Autodesk Inventor part; units mm, degrees
(part 5 of 5)
  arc A349 (-28.421, 226.0743) -> (-28.921, 225.5743) centre (-28.421, 225.5743) ccw
  arc A350 (-15.421, 212.0743) -> (-14.921, 212.5743) centre (-15.421, 212.5743) ccw
  arc A351 (-14.921, 225.5743) -> (-15.421, 226.0742) centre (-15.421, 225.5743) ccw
  line L356 (-28.921, 236.3868) -> (-28.921, 249.3868)
  line L357 (-14.921, 236.3868) -> (-14.921, 249.3868)
  line L358 (-28.421, 235.8868) -> (-15.421, 235.8868)
  line L359 (-28.421, 249.8868) -> (-15.421, 249.8867)
  arc A352 (-28.921, 236.3868) -> (-28.421, 235.8868) centre (-28.421, 236.3868) ccw
  arc A353 (-28.421, 249.8868) -> (-28.921, 249.3868) centre (-28.421, 249.3868) ccw
  arc A354 (-15.421, 235.8868) -> (-14.921, 236.3868) centre (-15.421, 236.3867) ccw
  arc A355 (-14.921, 249.3868) -> (-15.421, 249.8867) centre (-15.421, 249.3867) ccw
  line L360 (-28.921, 260.1993) -> (-28.921, 273.1993)
  line L361 (-14.921, 260.1992) -> (-14.921, 273.1993)
  line L362 (-28.421, 259.6993) -> (-15.421, 259.6993)
  line L363 (-28.421, 273.6992) -> (-15.421, 273.6992)
  arc A356 (-28.921, 260.1993) -> (-28.421, 259.6993) centre (-28.421, 260.1993) ccw
  arc A357 (-28.421, 273.6992) -> (-28.921, 273.1993) centre (-28.421, 273.1993) ccw
  arc A358 (-15.421, 259.6993) -> (-14.921, 260.1992) centre (-15.421, 260.1993) ccw
  arc A359 (-14.921, 273.1993) -> (-15.421, 273.6992) centre (-15.421, 273.1993) ccw
  line L364 (-28.921, 284.0118) -> (-28.921, 297.0118)
  line L365 (-14.921, 284.0118) -> (-14.921, 297.0118)
  line L366 (-28.421, 283.5118) -> (-15.421, 283.5118)
  line L367 (-28.421, 297.5118) -> (-15.421, 297.5118)
  arc A360 (-28.921, 284.0118) -> (-28.421, 283.5117) centre (-28.421, 284.0118) ccw
  arc A361 (-28.421, 297.5118) -> (-28.921, 297.0118) centre (-28.421, 297.0117) ccw
  arc A362 (-15.421, 283.5118) -> (-14.921, 284.0117) centre (-15.421, 284.0118) ccw
  arc A363 (-14.921, 297.0118) -> (-15.421, 297.5118) centre (-15.421, 297.0118) ccw
  line L368 (-28.921, 310.2055) -> (-28.921, 323.2055)
  line L369 (-14.921, 310.2055) -> (-14.921, 323.2055)
  line L370 (-28.421, 309.7055) -> (-15.421, 309.7055)
  line L371 (-28.421, 323.7055) -> (-15.421, 323.7055)
  arc A364 (-28.921, 310.2055) -> (-28.421, 309.7055) centre (-28.421, 310.2055) ccw
  arc A365 (-28.421, 323.7055) -> (-28.921, 323.2055) centre (-28.421, 323.2055) ccw
  arc A366 (-15.421, 309.7055) -> (-14.921, 310.2055) centre (-15.421, 310.2055) ccw
  arc A367 (-14.921, 323.2055) -> (-15.421, 323.7055) centre (-15.421, 323.2055) ccw
  line L372 (-28.921, 329.2555) -> (-28.921, 342.2555)
  line L373 (-14.921, 329.2555) -> (-14.921, 342.2555)
  line L374 (-28.421, 328.7555) -> (-15.421, 328.7555)
  line L375 (-28.421, 342.7555) -> (-15.421, 342.7555)
  arc A368 (-28.921, 329.2555) -> (-28.421, 328.7555) centre (-28.421, 329.2555) ccw
  arc A369 (-28.421, 342.7555) -> (-28.921, 342.2555) centre (-28.421, 342.2555) ccw
  arc A370 (-15.421, 328.7555) -> (-14.921, 329.2555) centre (-15.421, 329.2555) ccw
  arc A371 (-14.921, 342.2555) -> (-15.421, 342.7555) centre (-15.421, 342.2555) ccw
  line L376 (-28.921, 348.3055) -> (-28.921, 361.3055)
  line L377 (-14.921, 348.3055) -> (-14.921, 361.3055)
  line L378 (-28.421, 347.8055) -> (-15.421, 347.8055)
  line L379 (-28.421, 361.8055) -> (-15.421, 361.8055)
  arc A372 (-28.921, 348.3055) -> (-28.421, 347.8055) centre (-28.421, 348.3055) ccw
  arc A373 (-28.421, 361.8055) -> (-28.921, 361.3055) centre (-28.421, 361.3055) ccw
  arc A374 (-15.421, 347.8055) -> (-14.921, 348.3055) centre (-15.421, 348.3055) ccw
  arc A375 (-14.921, 361.3055) -> (-15.421, 361.8055) centre (-15.421, 361.3055) ccw
  line L380 (-12.396, 16.668) -> (-12.396, 364.3305)
  line L381 (-131.4585, 16.668) -> (-131.4585, 364.3305)
  line L382 (-12.396, 16.668) -> (-131.4585, 16.668)
  line L383 (-12.396, 364.3305) -> (-131.4585, 364.3305)
  point P0 (-71.9272, 364.3305)
  point P1 (-14.921, 28.5742)
  point P2 (-47.471, 269.2243)
  point P3 (-34.471, 269.2242)
  point P4 (-33.971, 269.7243)
  point P5 (-33.971, 282.7243)
  point P6 (-34.471, 283.2243)
  point P7 (-47.471, 283.2243)
  point P8 (-47.971, 282.7243)
  point P9 (-47.971, 269.7243)
  point P10 (-46.471, 260.7863)
  point P11 (-31.971, 261.2863)
  point P12 (-31.971, 267.2863)
  point P13 (-32.471, 267.7862)
  point P14 (-46.471, 267.7863)
  point P15 (-46.971, 267.2863)
  point P16 (-46.971, 261.2863)
  point P17 (-31.971, 285.1623)
  point P18 (-31.971, 291.1622)
  point P19 (-32.471, 291.6623)
  point P20 (-46.971, 285.1623)
  point P21 (-47.471, 328.7555)
  point P22 (-33.971, 329.2555)
  point P23 (-33.971, 342.2555)
  point P24 (-34.471, 342.7555)
  point P25 (-47.471, 342.7555)
  point P26 (-47.971, 342.2555)
  point P27 (-47.971, 329.2555)
  point P28 (-66.521, 273.9868)
  point P29 (-53.021, 274.4868)
  point P30 (-53.521, 287.9868)
  point P31 (-51.521, 265.5487)
  point P32 (-66.021, 266.0488)
  point P33 (-65.521, 289.4248)
  point P34 (-51.521, 289.4248)
  point P35 (-51.021, 295.9248)
  point P36 (-65.521, 296.4248)
  point P37 (-28.421, 259.6993)
  point P38 (-15.421, 259.6993)
  point P39 (-14.921, 273.1993)
  point P40 (-15.421, 273.6992)
  point P41 (-28.421, 273.6992)
  point P42 (-28.921, 273.1993)
  point P43 (-28.921, 260.1993)
  point P44 (-28.421, 283.5118)
  point P45 (-15.421, 283.5118)
  point P46 (-14.921, 297.0118)
  point P47 (-15.421, 297.5118)
  point P48 (-28.921, 297.0118)
  point P49 (-28.921, 284.0118)
  point P50 (-28.421, 309.7055)
  point P51 (-15.421, 309.7055)
  point P52 (-14.921, 310.2055)
  point P53 (-14.921, 323.2055)
  point P54 (-15.421, 323.7055)
  point P55 (-28.421, 323.7055)
  point P56 (-28.921, 323.2055)
  point P57 (-28.921, 310.2055)
  point P58 (-28.421, 328.7555)
  point P59 (-15.421, 328.7555)
  point P60 (-14.921, 329.2555)
  point P61 (-14.921, 342.2555)
  point P62 (-15.421, 342.7555)
  point P63 (-28.421, 342.7555)
  point P64 (-28.921, 342.2555)
  point P65 (-28.921, 329.2555)
  point P66 (-28.421, 347.8055)
  point P67 (-15.421, 347.8055)
  point P68 (-14.921, 348.3055)
  point P69 (-14.921, 361.3055)
  point P70 (-15.421, 361.8055)
  point P71 (-28.421, 361.8055)
  point P72 (-28.921, 361.3055)
  point P73 (-28.921, 348.3055)
  point P74 (-115.4335, 266.843)
  point P75 (-115.4335, 285.893)
  point P76 (-115.4335, 299.893)
  point P77 (-104.621, 276.368)
  point P78 (-91.621, 276.368)
  point P79 (-91.121, 289.868)
  point P80 (-104.621, 290.368)
  point P81 (-105.121, 289.868)
  point P82 (-105.121, 276.868)
  point P83 (-89.621, 267.93)
  point P84 (-89.121, 268.43)
  point P85 (-89.121, 274.43)
  point P86 (-104.121, 274.43)
  point P87 (-104.121, 268.43)
  point P88 (-89.621, 298.806)
  point P89 (-104.121, 298.306)
  point P90 (-104.621, 309.7055)
  point P91 (-91.621, 309.7055)
  point P92 (-91.121, 310.2055)
  point P93 (-91.121, 323.2055)
  point P94 (-91.621, 323.7055)
  point P95 (-91.121, 329.2555)
  point P96 (-91.121, 342.2555)
  point P97 (-91.621, 342.7555)
  point P98 (-104.621, 342.7555)
  point P99 (-105.121, 342.2555)
  point P100 (-105.121, 329.2555)
  point P101 (-104.621, 347.8055)
  point P102 (-91.621, 347.8055)
  point P103 (-91.121, 348.3055)
  point P104 (-91.121, 361.3055)
  point P105 (-91.621, 361.8055)
  point P106 (-104.621, 361.8055)
  point P107 (-105.121, 348.3055)
  point P108 (-85.571, 257.318)
  point P109 (-72.071, 257.818)
  point P110 (-72.071, 270.818)
  point P111 (-86.071, 270.818)
  point P112 (-86.071, 257.818)
  point P113 (-72.571, 281.1305)
  point P114 (-72.071, 281.6305)
  point P115 (-86.071, 281.6305)
  point P116 (-85.571, 309.7055)
  point P117 (-72.071, 310.2055)
  point P118 (-72.571, 323.7055)
  point P119 (-85.571, 323.7055)
  point P120 (-85.571, 328.7555)
  point P121 (-72.071, 329.2555)
  point P122 (-72.571, 342.7555)
  point P123 (-86.071, 342.2555)
  point P124 (-86.071, 329.2555)
  point P125 (-72.071, 348.3055)
  point P126 (-85.571, 361.8055)
  point P127 (-86.071, 361.3055)
  point P128 (-86.071, 348.3055)
  point P129 (-47.471, 195.4055)
  point P130 (-34.471, 195.4055)
  point P131 (-33.971, 195.9055)
  point P132 (-33.971, 208.9055)
  point P133 (-34.471, 209.4055)
  point P134 (-47.471, 209.4055)
  point P135 (-47.971, 208.9055)
  point P136 (-47.971, 195.9055)
  point P137 (-47.471, 214.4555)
  point P138 (-34.471, 214.4555)
  point P139 (-33.971, 214.9555)
  point P140 (-33.971, 227.9555)
  point P141 (-34.471, 228.4555)
  point P142 (-47.471, 228.4555)
  point P143 (-47.971, 227.9555)
  point P144 (-47.971, 214.9555)
  point P145 (-34.471, 233.5055)
  point P146 (-33.971, 234.0055)
  point P147 (-33.971, 247.0055)
  point P148 (-34.471, 247.5055)
  point P149 (-47.471, 247.5055)
  point P150 (-27.421, 194.1367)
  point P151 (-13.421, 194.1368)
  point P152 (-12.921, 194.6368)
  point P153 (-12.921, 200.6368)
  point P154 (-13.421, 201.1368)
  point P155 (-27.421, 201.1368)
  point P156 (-27.921, 200.6368)
  point P157 (-27.921, 194.6368)
  point P158 (-28.421, 212.0743)
  point P159 (-15.421, 212.0743)
  point P160 (-14.921, 212.5743)
  point P161 (-14.921, 225.5743)
  point P162 (-15.421, 226.0742)
  point P163 (-28.421, 226.0743)
  point P164 (-28.921, 225.5743)
  point P165 (-28.921, 212.5743)
  point P166 (-28.421, 235.8868)
  point P167 (-15.421, 235.8868)
  point P168 (-14.921, 236.3868)
  point P169 (-14.921, 249.3868)
  point P170 (-15.421, 249.8868)
  point P171 (-28.421, 249.8868)
  point P172 (-28.921, 249.3868)
  point P173 (-28.921, 236.3868)
  point P174 (-128.4335, 181.118)
  point P175 (-115.4335, 181.118)
  point P176 (-114.9335, 181.618)
  point P177 (-114.9335, 194.618)
  point P178 (-115.4335, 195.118)
  point P179 (-128.4335, 195.118)
  point P180 (-128.9335, 194.618)
  point P181 (-128.4335, 200.168)
  point P182 (-115.4335, 200.168)
  point P183 (-114.9335, 200.668)
  point P184 (-114.9335, 213.668)
  point P185 (-128.4335, 214.168)
  point P186 (-128.9335, 200.668)
  point P187 (-115.4335, 228.743)
  point P188 (-114.9335, 229.243)
  point P189 (-114.9335, 242.243)
  point P190 (-128.4335, 247.793)
  point P191 (-115.4335, 247.793)
  point P192 (-128.4335, 261.793)
  point P193 (-128.9335, 248.293)
  point P194 (-91.121, 261.293)
  point P195 (-91.621, 261.793)
  point P196 (-104.621, 261.793)
  point P197 (-105.121, 261.293)
  point P198 (-53.521, 185.8805)
  point P199 (-53.021, 186.3805)
  dimension "d74" = 14.921
  dimension "d75" = 16.668
  constraints: 2 other
  measures "d74" distance from line of L2 point (-14.921, 28.574)
extrude "Extrusion3" cut sketch "Sketch5" against normal blind 2 contours L4 A1 L7 A3 L5 A2 L6 A0 | L8 A5 L11 A7 L9 A6 L10 A4 | L12 A9 L15 A11 L13 A10 L14 A8 | L16 A13 L19 A15 L17 A14 L18 A12 | L20 A17 L23 A19 L21 A18 L22 A16 | L24 A21 L27 A23 L25 A22 L26 A20 | L28 A25 L31 A27 L29 A26 L30 A24 | L32 A29 L35 A31 L33 A30 L34 A28 | L36 A33 L39 A35 L37 A34 L38 A32 | L40 A37 L43 A39 L41 A38 L42 A36 | L44 A41 L47 A43 L45 A42 L46 A40 | L48 A45 L51 A47 L49 A46 L50 A44 | L52 A49 L55 A51 L53 A50 L54 A48 | L56 A53 L59 A55 L57 A54 L58 A52 | L60 A57 L63 A59 L61 A58 L62 A56 | L64 A61 L67 A63 L65 A62 L66 A60 | L68 A65 L71 A67 L69 A66 L70 A64 | L72 A69 L75 A71 L73 A70 L74 A68 | L76 A73 L79 A75 L77 A74 L78 A72 | L80 A77 L83 A79 L81 A78 L82 A76 | L84 A81 L87 A83 L85 A82 L86 A80 | L88 A85 L91 A87 L89 A86 L90 A84 | L92 A89 L95 A91 L93 A90 L94 A88 | L96 A93 L99 A95 L97 A94 L98 A92 | L100 A97 L103 A99 L101 A98 L102 A96 | L104 A101 L107 A103 L105 A102 L106 A100 | L108 A105 L111 A107 L109 A106 L110 A104 | L112 A109 L115 A111 L113 A110 L114 A108 | L116 A113 L119 A115 L117 A114 L118 A112 | L120 A117 L123 A119 L121 A118 L122 A116 | L124 A121 L127 A123 L125 A122 L126 A120 | L128 A125 L131 A127 L129 A126 L130 A124 | L132 A129 L135 A131 L133 A130 L134 A128 | L136 A133 L139 A135 L137 A134 L138 A132 | L140 A137 L143 A139 L141 A138 L142 A136 | L144 A141 L147 A143 L145 A142 L146 A140 | L148 A145 L151 A147 L149 A146 L150 A144 | L152 A149 L155 A151 L153 A150 L154 A148 | L156 A153 L159 A155 L157 A154 L158 A152 | L160 A157 L163 A159 L161 A158 L162 A156 | L164 A161 L167 A163 L165 A162 L166 A160 | L168 A165 L171 A167 L169 A166 L170 A164 | L172 A169 L175 A171 L173 A170 L174 A168 | L176 A173 L179 A175 L177 A174 L178 A172 | L180 A177 L183 A179 L181 A178 L182 A176 | L184 A181 L187 A183 L185 A182 L186 A180 | L188 A185 L191 A187 L189 A186 L190 A184 | L192 A189 L195 A191 L193 A190 L194 A188 | L196 A193 L199 A195 L197 A194 L198 A192 | L200 A197 L203 A199 L201 A198 L202 A196 | L204 A201 L207 A203 L205 A202 L206 A200 | L208 A205 L211 A207 L209 A206 L210 A204 | L212 A209 L215 A211 L213 A210 L214 A208 | L216 A213 L219 A215 L217 A214 L218 A212 | L220 A217 L223 A219 L221 A218 L222 A216 | L224 A221 L227 A223 L225 A222 L226 A220 | L228 A225 L231 A227 L229 A226 L230 A224 | L232 A229 L235 A231 L233 A230 L234 A228 | L236 A233 L239 A235 L237 A234 L238 A232 | L240 A237 L243 A239 L241 A238 L242 A236 | L244 A241 L247 A243 L245 A242 L246 A240 | L248 A245 L251 A247 L249 A246 L250 A244 | L252 A249 L255 A251 L253 A250 L254 A248 | L256 A253 L259 A255 L257 A254 L258 A252 | L260 A257 L263 A259 L261 A258 L262 A256 | L264 A261 L267 A263 L265 A262 L266 A260 | L268 A265 L271 A267 L269 A266 L270 A264 | L272 A269 L275 A271 L273 A270 L274 A268 | L276 A273 L279 A275 L277 A274 L278 A272 | L280 A277 L283 A279 L281 A278 L282 A276 | L284 A281 L287 A283 L285 A282 L286 A280 | L288 A285 L291 A287 L289 A286 L290 A284 | L292 A289 L295 A291 L293 A290 L294 A288 | L296 A293 L299 A295 L297 A294 L298 A292 | L300 A297 L303 A299 L301 A298 L302 A296 | L304 A301 L307 A303 L305 A302 L306 A300 | L308 A305 L311 A307 L309 A306 L310 A304 | L312 A309 L315 A311 L313 A310 L314 A308 | L316 A313 L319 A315 L317 A314 L318 A312 | L320 A317 L323 A319 L321 A318 L322 A316 | L324 A321 L327 A323 L325 A322 L326 A320 | L328 A325 L331 A327 L329 A326 L330 A324 | L332 A329 L335 A331 L333 A330 L334 A328 | L336 A333 L339 A335 L337 A334 L338 A332 | L340 A337 L343 A339 L341 A338 L342 A336 | L344 A341 L347 A343 L345 A342 L346 A340 | L348 A345 L351 A347 L349 A346 L350 A344 | L352 A349 L355 A351 L353 A350 L354 A348 | L356 A353 L359 A355 L357 A354 L358 A352 | L360 A357 L363 A359 L361 A358 L362 A356 | L364 A361 L367 A363 L365 A362 L366 A360 | L368 A365 L371 A367 L369 A366 L370 A364 | L372 A369 L375 A371 L373 A370 L374 A368 | L376 A373 L379 A375 L377 A374 L378 A372
sketch "Sketch6" plane through (0, 2, 0) normal (0, 1, 0) x (1, 0, 0)
  line L0 (-139.621, 309.4231) -> (-111.121, 309.4231)
  line L1 (-111.121, 309.4231) -> (-111.121, 365.4231)
  line L2 (-111.121, 365.4231) -> (-139.621, 365.4231)
  line L3 (-139.621, 365.4231) -> (-139.621, 309.4231)
  line L4 (-105.121, 310.2055) -> (-105.121, 323.2055) projected
  point P0 (0, 0)
  dimension "d78" = 28.5
  dimension "d79" = 56
  dimension "d80" = 6
  constraints: 8 end point, 2 parallel, 1 horizontal, 1 perpendicular
  measures "d78" distance of L2.end L1.end
  measures "d79" distance of L1.end L0.end
  measures "d80" distance between parallel lines of L1 L4
body "Solid1"
